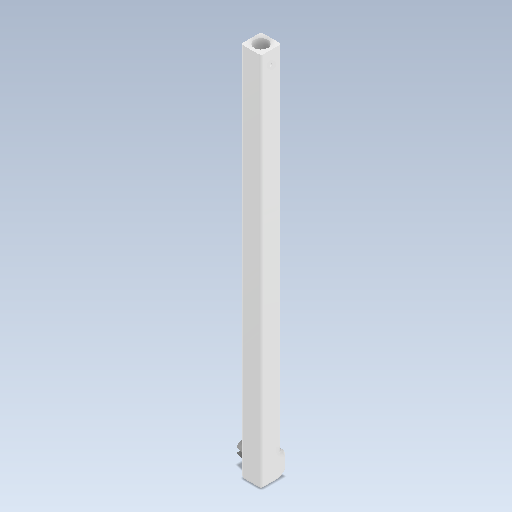
# Autodesk Inventor part: Eslabón conector M2
Saved by Autodesk Inventor 2021 (Build 250183000, 183)
## iProperties
Created: 2023-08-11
Part Number: Eslabón conector M2
Material: Plástico PPS
Document SubType Name: Modeling
Designer: Sergio
Density: 1.637 g/cm^3
Appearance: Suave - Blanco
Author: Sergio
Autodesk Inventor part; units mm, degrees
ref_plane "YZ Plane" through (0, 0, 0) normal (1, 0, 0) x (0, 1, 0)
ref_plane "XY Plane" through (0, 0, 0) normal (0, 0, 1) x (1, 0, 0)
sketch "Boceto1" plane through (0, 0, 0) normal (1, 0, 0) x (0, 1, 0)
  circle A0 centre (0, 0) radius 5
  line L0 (0, 0) -> (0, 6)
  line L1 (0, 6) -> (-4, 6)
  line L2 (-5, 5) -> (-5, 0)
  line L3 (0, 6) -> (181.05, 6)
  line L4 (181.05, 6) -> (187.5, 6)
  line L5 (187.5, 6) -> (189.65, 6)
  line L6 (190.65, 5) -> (190.65, -1)
  line L7 (189.65, -2) -> (4.5826, -2)
  arc A1 (-4, 6) -> (-5, 5) centre (-4, 5) ccw
  arc A2 (190.65, 5) -> (189.65, 6) centre (189.65, 5) ccw
  arc A3 (189.65, -2) -> (190.65, -1) centre (189.65, -1) ccw
  line L8 (3.5707, -3.5) -> (-3.5707, -3.5)
  point P0 (-5, 6)
  point P1 (190.65, 6)
  point P2 (190.65, -2)
  dimension "d0" = 10
  dimension "d1" = 6
  dimension "d2" = 5
  dimension "d3" = 181.05
  dimension "d4" = 6.45
  dimension "d5" = 3.15
  dimension "d6" = 8
  dimension "d7" = 1
  dimension "d8" = 1
  dimension "d45" = 1.5
  constraints: 18 end point, 10 point on circle, 9 point on line, 7 tangent, 4 centre point, 3 perpendicular, 1 coincident, 1 equal radius, 1 horizontal, 1 vertical
  measures "d0" diameter of A0
  measures "d1" distance of L0.start L0.end
  measures "d2" distance of L0.end point (-5, 6)
  measures "d3" distance of L0.end L3.end
  measures "d4" distance of L3.end L4.end
  measures "d5" distance of L4.end point (190.65, 6)
  measures "d6" distance of point (190.65, 6) point (190.65, -2)
  measures "d7" radius of A1
  measures "d8" radius of A2
  measures "d45" distance between parallel lines of L7 L8
extrude "Extrusión1" add sketch "Boceto1" along normal mid plane 8 contours A0 L8 | L2 A1 L1 L0 A0 | L0 L3 L4 L5 A2 L6 A3 L7 A0 picked at (0, -0.6667)
fillet "Empalme1" radius 1 18 edges at (-4, 190.3571, 5.7071) (-4, 190.65, 2) (-4, 190.3571, -1.7071) (-4, 97.1163, -2) (-4, -4.7071, 5.7071) (-4, -5, 2.5) (-4, -4.6289, -1.8903) (-4, 4.1451, -2.7962) (-4, 92.825, 6) (4, -4.7071, 5.7071) (4, -5, 2.5) (4, -4.6289, -1.8903) (4, 4.1451, -2.7962) (4, 190.3571, 5.7071) (4, 190.65, 2) (4, 190.3571, -1.7071) (4, 97.1163, -2) (4, 92.825, 6)
sketch "Boceto2" plane through (-4, 0, 0) normal (-1, 0, 0) x (0, 0, 1)
  circle A0 centre (0, 0) radius 5.5
  line L0 (4.7631, 2.75) -> (-2, 14.4641)
  line L1 (-2, 189.65) -> (-2, 4.5826) projected
  line L2 (5.5, 0) -> (5.5, -5.5)
  line L3 (0, -5) -> (5, -5) projected
  line L4 (0, -5.5) -> (5.5, -5.5)
  line L5 (-2, 14.4641) -> (-2, 5.1235)
  dimension "d12" = 11
  dimension "d13" = 30
  constraints: 8 end point, 4 point on circle, 2 perpendicular, 2 point on line, 1 centre point, 1 coincident, 1 tangent
  measures "d12" diameter of A0
  measures "d13" angle of L1 L0
extrude "Extrusión2" cut sketch "Boceto2" against normal blind 2.5
sketch "Boceto3" plane through (0, 0, 0) normal (0, 0, 1) x (1, 0, 0)
  line L0 (-3, 190.65) -> (3, 190.65) projected
  line L1 (0, 190.65) -> (0, 181.05)
  line L2 (1.4, 190.65) -> (1.4, 181.05)
  line L3 (-1.4, 190.65) -> (-1.4, 181.05)
  line L4 (1.4, 190.65) -> (-1.4, 190.65)
  line L5 (0, 181.05) -> (1.4, 181.05)
  line L6 (0, 181.05) -> (-1.4, 181.05)
  point P0 (0, 0)
  dimension "d16" = 9.6
  dimension "d17" = 1.4
  dimension "d18" = 1.4
  constraints: 12 end point, 2 parallel, 1 midpoint, 1 perpendicular, 1 point on line, 1 vertical
  measures "d16" distance of L1.start L1.end
  measures "d17" distance between parallel lines of L1 L2
  measures "d18" distance between parallel lines of L1 L3
extrude "Extrusión3" cut sketch "Boceto3" along normal mid plane 16
fillet "Empalme4" radius 1 2 edges at (-1.4, 181.05, 2) (1.4, 181.05, 2)
sketch "Boceto11" plane through (0, 0, 0) normal (1, 0, 0) x (0, 1, 0)
  line L0 (0, 0) -> (0, 6)
  line L1 (0, 6) -> (181.05, 6)
  line L2 (189.65, 6) -> (-4, 6) projected
  line L3 (181.05, 6) -> (187.5, 6)
  line L4 (187.5, 6) -> (187.5, 0.55)
  circle A0 centre (187.5, 0.55) radius 1.15
  dimension "d66" = 6
  dimension "d67" = 181.05
  dimension "d68" = 6.45
  dimension "d69" = 5.45
  dimension "d70" = 2.3
  constraints: 8 end point, 2 point on line, 1 centre point, 1 coincident, 1 perpendicular, 1 vertical
  measures "d66" distance of L0.start L0.end
  measures "d67" distance of L0.end L1.end
  measures "d68" distance of L1.end L3.end
  measures "d69" distance of L3.end L4.end
  measures "d70" diameter of A0
extrude "Extrusión9" cut sketch "Boceto11" along normal through all both and the other way through all
sketch "Boceto6" plane through (0, 0, 0) normal (0, 0, 1) x (1, 0, 0)
  line L0 (0, 0) -> (-1.5, 0)
  line L1 (-1.5, 0) -> (-1.5, -3)
  line L2 (-1.5, -5) -> (-1.5, 4.5826) projected
  line L3 (-1.5, -3) -> (-4.5, -3)
  line L4 (-1.5, 0) -> (-9.5, 0)
  line L5 (-4.5, -3) -> (-4.5, -3.5)
  line L6 (-9.5, 0) -> (-9.5, -2.3732)
  line L7 (-9.5, -2.3732) -> (-4.5, -3.5)
  dimension "d27" = 1.5
  dimension "d28" = 3
  dimension "d29" = 3
  dimension "d30" = 8
  dimension "d31" = 0.5
  dimension "d32" = 2.3732
  constraints: 14 end point, 3 horizontal, 2 vertical, 1 point on line
  measures "d27" distance of L0.start L0.end
  measures "d28" distance of L0.end L1.end
  measures "d29" distance of L1.end L3.end
  measures "d30" distance of L0.end L4.end
  measures "d31" distance of L3.end L5.end
  measures "d32" distance of L4.end L6.end
revolve "Revolución1" add sketch "Boceto6" angle 360 about axis through (-1.5, 0, 0) along (-1, 0, 0)
sketch "Boceto7" plane through (0, 0, 0) normal (0, 0, 1) x (1, 0, 0)
  line L0 (0, 0) -> (-1.5, 0)
  line L1 (-1.5, 0) -> (-4.5, 0)
  line L2 (-4.5, 0) -> (-9.5, 0)
  line L3 (-9.5, 0) -> (-9.5, -1)
  line L4 (-9.5, 2.3732) -> (-9.5, -2.3732) projected
  line L5 (-9.5, -1) -> (-2.5, -1)
  line L6 (-2.5, -1) -> (-2.5, 1)
  line L7 (-2.5, 1) -> (-9.5, 1)
  line L8 (-9.5, 1) -> (-9.5, 0)
  point P0 (-9.5, 1)
  dimension "d34" = 1.5
  dimension "d35" = 3
  dimension "d36" = 5
  dimension "d37" = 1
  dimension "d38" = 7
  dimension "d39" = 2
  constraints: 16 end point, 4 perpendicular, 4 point on line, 1 horizontal
  measures "d34" distance of L0.start L0.end
  measures "d35" distance of L0.end L1.end
  measures "d36" distance of L1.end L2.end
  measures "d37" distance of L2.end L3.end
  measures "d38" distance of L3.end L5.end
  measures "d39" distance of L5.end L6.end
extrude "Extrusión5" cut sketch "Boceto7" along normal mid plane 7
fillet "Empalme2" radius 1 2 edges at (-2.5, -1, 0) (-2.5, 1, 0)
ref_plane "Plano de trabajo2" through (0, 177.05, 0) normal (0, 1, 0) x (-1, 0, 0)
sketch "Boceto8" plane through (0, 177.05, 0) normal (0, 1, 0) x (-1, 0, 0)
  line L0 (0, 0) -> (0, 2)
  line L1 (16, 18) -> (-16, 18)
  line L2 (-16, 18) -> (-16, -14)
  line L3 (-16, -14) -> (16, -14)
  line L4 (16, -14) -> (16, 18)
  line L5 (16, 18) -> (-16, -14) construction
  line L6 (-16, 18) -> (16, -14) construction
  point P0 (0, 0)
  dimension "d49" = 2
  dimension "d50" = 32
  dimension "d51" = 32
  dimension "d78" = 0
  constraints: 14 end point, 2 midpoint, 2 parallel, 1 horizontal, 1 perpendicular
  measures "d49" distance of L0.start L0.end
  measures "d50" distance of L3.end L2.end
  measures "d51" distance of L2.end L1.end
  measures "d78" distance of point (0, 0) L0.start
extrude "Extrusión6" cut sketch "Boceto8" against normal blind 34
sketch "Boceto9" plane through (0, 177.05, 0) normal (0, -1, 0) x (-1, 0, 0)
  line L0 (3, -6) -> (-3, -6) projected
  line L1 (0, 0) -> (0, -2)
  circle A0 centre (0, -2) radius 2.75
  point P0 (0, 0)
  point P1 (-2.6, -6)
  dimension "d55" = 2
  dimension "d56" = 5.5
  dimension "d79" = 0
  dimension "d80" = 0
  constraints: 2 end point, 1 centre point, 1 vertical
  measures "d55" distance of L1.start L1.end
  measures "d56" diameter of A0
  measures "d79" distance of point (0, 0) L1.start
  measures "d80" distance of L1.end A0.centre
extrude "Extrusión7" cut sketch "Boceto9" along normal blind 44.2
sketch "Boceto10" plane through (0, 177.05, 0) normal (0, -1, 0) x (-1, 0, 0)
  circle A0 centre (0, -2) radius 2.6 projected
  circle A1 centre (0, -2) radius 3
  point P0 (0, 0)
  dimension "d59" = 6
  constraints: 1 centre point, 1 coincident
  measures "d59" diameter of A1
extrude "Extrusión8" [suppressed]
fillet "Empalme3" [suppressed]
sketch "Boceto13" plane through (0, 143.05, 0) normal (0, 1, 0) x (1, 0, 0)
  line L0 (16, -16) -> (-16, -16)
  line L1 (-16, -16) -> (-16, 16)
  line L2 (-16, 16) -> (16, 16)
  line L3 (16, 16) -> (16, -16)
  line L4 (16, -16) -> (-16, 16) construction
  line L5 (-16, -16) -> (16, 16) construction
  point P0 (0, 0)
  dimension "d81" = 32
  dimension "d82" = 32
  constraints: 12 end point, 2 midpoint, 2 parallel, 1 horizontal, 1 perpendicular
  measures "d81" distance of L1.end L2.end
  measures "d82" distance of L0.end L1.end
extrude "Extrusión10" cut sketch "Boceto13" along normal blind 181.05
sketch "Boceto14" plane through (0, 0, 0) normal (1, 0, 0) x (0, 1, 0)
  line L0 (0, 0) -> (0, 6)
  line L1 (0, 6) -> (137.85, 6)
  line L2 (137.85, 6) -> (137.85, 2)
  circle A0 centre (137.85, 2) radius 0.5
  dimension "d85" = 6
  dimension "d86" = 137.85
  dimension "d87" = 4
  dimension "d88" = 1
  constraints: 6 end point, 2 vertical, 1 centre point, 1 coincident, 1 perpendicular
  measures "d85" distance of L0.start L0.end
  measures "d86" distance of L0.end L1.end
  measures "d87" distance of L1.end L2.end
  measures "d88" diameter of A0
extrude "Extrusión11" cut sketch "Boceto14" along normal through all both and the other way through all
equation "\"d0\" = width_r3"
equation "\"d1\" = 0.5 * width_r3 + offset"
equation "\"d2\" = 0.5 * width_r3"
equation "\"d3\" = lenght_body_link - 0.5 * width_r3"
equation "\"d4\" = shaft_y"
equation "\"d5\" = 0.5 * Djoint_shaft + 2 * offset"
equation "\"d6\" = width_link"
equation "\"d45\" = 1.5 * offset"
equation "\"d9\" = width_link"
equation "\"d12\" = width_r3 + offset"
equation "\"d14\" = 0.5 * width_link - 0.5 * t_thikness"
equation "\"d16\" = 0.5 * Djoint_shaft + 2 * offset + shaft_y"
equation "\"d17\" = 0.25 * offset + 0.5 * wire_D"
equation "\"d18\" = 0.25 * offset + 0.5 * wire_D"
equation "\"d19\" = 2 * width_link"
equation "\"d63\" = offset"
equation "\"d27\" = 0.5 * t_thikness"
equation "\"d28\" = 0.5 * sj_diam_shaft"
equation "\"d29\" = t_thikness"
equation "\"d30\" = t_thikness + sj_head_height"
equation "\"d31\" = 0.5 * sj_head_D - 0.5 * sj_diam_shaft"
equation "\"d32\" = 0.5 * sj_head_d"
equation "\"d34\" = 0.5 * t_thikness"
equation "\"d35\" = t_thikness"
equation "\"d36\" = sj_head_height"
equation "\"d37\" = 0.5 * sj_groove"
equation "\"d38\" = sj_groove_deep"
equation "\"d39\" = sj_groove"
equation "\"d40\" = sj_head_D"
equation "\"d46\" = 0.5 * sj_groove"
equation "\"d52\" = spring_lenght + 3 * thikness"
equation "\"d59\" = spring_int_d"
equation "\"d60\" = thikness"
equation "\"d62\" = offset"
equation "\"offset\" = 1"
equation "\"wire_D\" = 2.3"
equation "\"width_link\" = 8"
equation "\"Djoint_shaft\" = 2.3"
equation "\"shaft_x\" = 1.45"
equation "\"shaft_y\" = 6.45"
equation "\"lenght_body_link\" = 186.05"
equation "\"m2_theta3f\" = -60deg"
equation "\"width_r3\" = 10"
equation "\"t_thikness\" = 3"
equation "\"sj_diam_shaft\" = 6"
equation "\"sj_groove\" = 2"
equation "\"sj_groove_deep\" = 7"
equation "\"sj_head_D\" = 7"
equation "\"sj_head_d\" = 4.7464"
equation "\"sj_head_height\" = 5"
equation "\"thikness\" = 2"
equation "\"spring_int_d\" = 6"
equation "\"spring_lenght\" = 28"
equation "\"r1\" = 5.55"
equation "\"r2o\" = 59.75"
equation "\"delta_y\" = 6"
equation "\"wire_d\" = 1"
equation "\"width_ang_spring\" = 5"
equation "\"spring_int_diam\" = 8.5"
equation "\"spring_ext_diam\" = 10.5"
equation "\"r3\" = 8.25"
equation "\"r3R\" = 4.75"
equation "\"r3T\" = 6.74537"
equation "\"alpha\" = 54.847297deg"
equation "\"alpha2\" = 270deg"
equation "\"theta3_recogido\" = 305.152703deg"
equation "\"delta_theta_3\" = 45deg"
equation "\"joint_width\" = 12"
equation "\"joint_radius\" = 7.75"
equation "\"shaft_width\" = 15"
equation "\"shaft_joint_diameter\" = 7.75"
equation "\"separation_space\" = 0.5"
equation "\"height_finger\" = 42"
equation "\"cell_screw_head_diameter\" = 4"
equation "\"cell_screw_diameter\" = 2"
equation "\"cell_space\" = 2"
equation "\"cell_width\" = 6"
equation "\"cell_theta_position\" = 60deg"
equation "\"cell_thikness\" = 1"
equation "\"cell_lenght\" = 37"
equation "\"cell_z_space\" = 5"
equation "\"Dt\" = 1.05949"
equation "\"lenght_bar_support\" = 201.65"
equation "\"wire_spring_d\" = 1"
equation "\"trigger_offset\" = 2"
equation "\"m2_theta2o\" = 107deg"
equation "\"m2_r2\" = 28"
equation "\"e\" = 9"
equation "\"So\" = 17"
equation "\"m2_theta3o\" = -30deg"
equation "\"m2_r3\" = 19.75"
equation "\"m2_delta_theta1\" = 15deg"
equation "\"trigger_thumb_lenght\" = 6"
equation "\"width_r12\" = 8"
equation "\"m2_r1\" = 25.2"
equation "\"r3_thikness\" = 3.5"
equation "\"tg_width\" = 4"
equation "\"pivot_screw_d\" = 4"
equation "\"pivot_diameter\" = 7"
equation "\"sf_lenght\" = 9.5"
equation "\"sf_base\" = 3"
equation "\"sf_head_height\" = 3"
equation "\"sf_head_width\" = 4.5"
equation "\"sf_head_offset\" = 0.25"
equation "\"sf_head_grip_width\" = 2"
equation "\"sf_head_angle\" = 45deg"
equation "\"sf_thikness\" = 5"
equation "\"screw_Dhead\" = 8"
equation "\"screw_d\" = 4"
equation "\"screw_lenght\" = 12"
equation "\"screwJ_base_D\" = 9"
equation "\"screwJ_top_D\" = 13"
equation "\"gj_D\" = 6"
equation "\"gj_d\" = 4"
equation "\"gj_out_section\" = 6"
equation "\"agarradera_theta\" = 60deg"
equation "\"agarradera_width\" = 4"
equation "\"sfbox_theta1\" = 60deg"
equation "\"sfbox_theta2\" = 45deg"
equation "\"position\" = 39.13077"
equation "\"fat_width_slider\" = 2"
equation "\"sfbox_tip_width\" = 2.5"
equation "\"flex_separation_theta\" = 60deg"
equation "\"sf_flex_separation\" = 38.66667"
equation "\"ext_width_slider\" = 3.5"
equation "\"sf_box_width\" = 1.5"
equation "\"slim_width_slider\" = 1.5"
equation "\"sfbox_width\" = 1.5"
equation "\"int_width_slider\" = 2"
equation "\"box_fat_slider_lenght\" = 67"
equation "\"box_slim_slider_lenght\" = 116"
equation "\"thikness_box\" = 1.5"
equation "\"box_in_height\" = 35"
equation "\"box_in_width\" = 72"
equation "\"box_in_deep\" = 77"
equation "\"agarradera_position\" = 82.13077"
